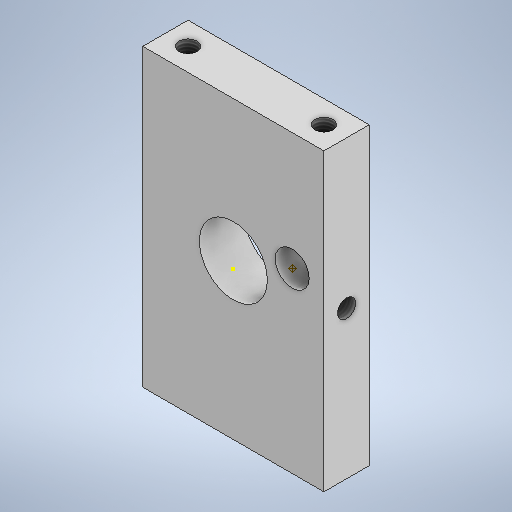
# Autodesk Inventor part: Rb PEEK - Corto con ventana
Saved by Autodesk Inventor 2025.3 (Build 293356000, 356)
## iProperties
Created: 2025-05-09
Part Number: Rb PEEK - Corto con ventana
Material: Generic
Document SubType Name: Modeling
Designer: E. Moreno
Density: 1 g/cm^3
Appearance: Default
Author: E. Moreno
Title: Rb PEEK - Corto con ventana
Autodesk Inventor part; units mm, degrees
ref_plane "YZ Plane" through (0, 0, 0) normal (1, 0, 0) x (0, 1, 0)
ref_plane "XZ Plane" through (0, 0, 0) normal (0, 1, 0) x (-1, 0, 0)
ref_plane "XY Plane" through (0, 0, 0) normal (0, 0, 1) x (1, 0, 0)
sketch "Sketch1" plane through (0, 0, 0) normal (0, 0, 1) x (1, 0, 0)
  line L0 (-20, -32.6) -> (20, -32.6)
  line L1 (20, -32.6) -> (20, 32.6)
  line L2 (20, 32.6) -> (-20, 32.6)
  line L3 (-20, 32.6) -> (-20, -32.6)
  line L4 (-20, -32.6) -> (20, 32.6) construction
  line L5 (20, -32.6) -> (-20, 32.6) construction
  point P0 (0, 0)
  dimension "d0" = 40
  dimension "d1" = 65.2
  constraints: 12 end point, 2 midpoint, 2 parallel, 1 horizontal, 1 perpendicular
  measures "d0" distance of L2.end L1.end
  measures "d1" distance of L1.end L0.end
extrude "Extrusion1" add sketch "Sketch1" along normal blind 10
sketch "Sketch2" plane through (-20, 32.6, 0) normal (0, 1, 0) x (1, 0, 0)
  line L0 (40, -10) -> (40, -5)
  line L1 (40, 0) -> (40, -10) projected
  line L2 (40, -5) -> (35, -5)
  circle A0 centre (35, -5) radius 2
  line L3 (20, 0) -> (20, -10)
  circle A1 centre (5, -5) radius 2
  dimension "d4" = 5
  dimension "d5" = 5
  dimension "d6" = 4
  constraints: 6 end point, 2 centre point, 2 coincident, 2 symmetric about line, 1 midpoint, 1 perpendicular, 1 vertical, 1 other
  measures "d4" distance of L0.start L0.end
  measures "d5" distance of L0.end L2.end
  measures "d6" diameter of A0
extrude "Extrusion2" cut sketch "Sketch2" against normal blind 25
mirror "Mirror1" about plane through (0, 0, 0) normal (0, 1, 0) of "Extrusion2"
thread "Thread1" size "M4x0.7" class "6H" standard "ANSI Metric M Profile" full length
thread "Thread2" size "M4x0.7" class "6H" standard "ANSI Metric M Profile" full length
thread "Thread3" size "M4x0.7" class "6H" standard "ANSI Metric M Profile" full length
thread "Thread4" size "M4x0.7" class "6H" standard "ANSI Metric M Profile" full length
sketch "Sketch3" plane through (20, -32.6, 0) normal (1, 0, 0) x (0, 0, -1)
  line L0 (0, 32.6) -> (-5, 32.6)
  circle A0 centre (-5, 32.6) radius 2
  dimension "d17" = 5
  dimension "d18" = 4
  constraints: 2 end point, 1 centre point, 1 coincident, 1 horizontal
  measures "d17" distance of L0.start L0.end
  measures "d18" diameter of A0
extrude "Extrusion3" cut sketch "Sketch3" against normal blind 10
mirror "Mirror2" about plane through (0, 0, 0) normal (1, 0, 0) of "Extrusion3"
sketch "Sketch4" plane through (0, 0, 10) normal (0, 0, 1) x (1, 0, 0)
  point P0 (0, 0)
sketch "Sketch5" plane through (0, 0, 10) normal (0, 0, 1) x (1, 0, 0)
  line L0 (-20, -32.6) -> (20, -32.6) projected
  line L1 (0, -32.6) -> (0, 1.6)
  circle A0 centre (0, 1.6) radius 7.5
  line L2 (0, 1.6) -> (13, 1.6)
  line L3 (13, 1.6) -> (13, 6.6)
  circle A1 centre (13, 6.6) radius 3.75
  point P0 (0, 0)
  dimension "d21" = 34.2
  dimension "d22" = 15
  dimension "d29" = 13
  dimension "d33" = 5
  dimension "d34" = 7.5
  constraints: 6 end point, 3 coincident, 2 centre point, 2 vertical, 1 horizontal, 1 midpoint
  measures "d21" distance of L1.start L1.end
  measures "d22" diameter of A0
  measures "d29" distance of L2.start L2.end
  measures "d33" distance of L3.start L3.end
  measures "d34" diameter of A1
thread "Thread5" size "M4x0.7" class "6H" standard "ANSI Metric M Profile" full length
thread "Thread6" size "M4x0.7" class "6H" standard "ANSI Metric M Profile" full length
extrude "Extrusion6" cut sketch "Sketch5" against normal blind 10
sketch "Sketch6" plane through (0, 0, 10) normal (0, 0, 1) x (1, 0, 0)
  circle A0 centre (13, 6.6) radius 3.75 projected
body "Solid1"
